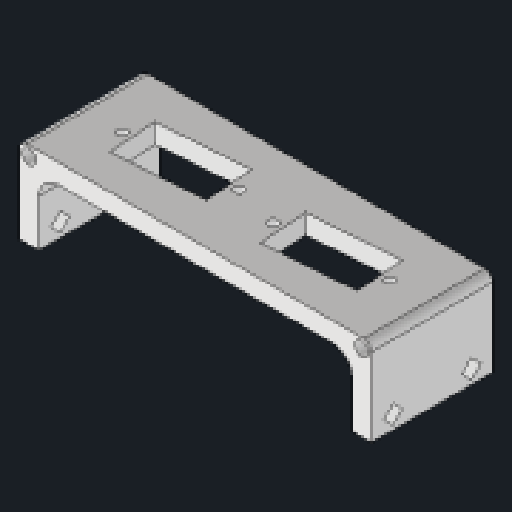
# Autodesk Inventor part: Module Frame
Saved by Autodesk Inventor 2023.2 (Build 272271030, 271C)
## iProperties
Created: 2024-02-26
Part Number: Module Frame
Material: Generic
Document SubType Name: Modeling
Designer: robpl
Density: 1 g/cm^3
Appearance: Default
Author: robpl
Autodesk Inventor part; units mm, degrees
ref_plane "YZ Plane" through (0, 0, 0) normal (1, 0, 0) x (0, 1, 0)
ref_plane "XZ Plane" through (0, 0, 0) normal (0, 1, 0) x (-1, 0, 0)
ref_plane "XY Plane" through (0, 0, 0) normal (0, 0, 1) x (1, 0, 0)
sketch "Sketch1" plane through (0, 0, 0) normal (0, 0, 1) x (1, 0, 0)
  line L0 (-40, 0) -> (40, 0)
  line L1 (40, 0) -> (40, 5)
  line L2 (40, 5) -> (-40, 5)
  line L3 (-40, 5) -> (-40, 0)
  line L4 (-40, 5) -> (-45, 5)
  line L5 (-45, 5) -> (-45, -17)
  line L6 (-45, -17) -> (-40, -17)
  line L7 (-40, -17) -> (-40, 5)
  line L8 (40, 5) -> (45, 5)
  line L9 (45, 5) -> (45, -17)
  line L10 (45, -17) -> (40, -17)
  line L11 (40, -17) -> (40, 5)
  point P0 (0, 0)
  point P1 (0, 0)
  point P2 (40, 0)
  dimension "d0" = 5
  dimension "d1" = 80
  dimension "d2" = 22
  dimension "d11" = 5
  constraints: 24 end point, 6 parallel, 3 horizontal, 3 perpendicular, 2 equal length, 1 coincident, 1 midpoint
  measures "d0" distance of L0.end L1.end
  measures "d1" distance of L0.start L0.end
  measures "d2" distance of L6.end L2.end
  measures "d11" distance of L9.end L10.end
extrude "Extrusion1" add sketch "Sketch1" along normal mid plane 32
sketch "Sketch2" plane through (45, -17, -16) normal (1, 0, 0) x (0, 0, -1)
  line L0 (-28.4042, 3.5) -> (-26, 1.0958)
  line L1 (-26, 1.0958) -> (-23.5958, 3.5)
  line L2 (-23.5958, 3.5) -> (-26, 5.9042)
  line L3 (-26, 5.9042) -> (-28.4042, 3.5)
  line L4 (-28.4042, 3.5) -> (-23.5958, 3.5) construction
  line L5 (-26, 1.0958) -> (-26, 5.9042) construction
  line L6 (-8.4042, 3.5) -> (-6, 1.0958)
  line L7 (-6, 1.0958) -> (-3.5958, 3.5)
  line L8 (-3.5958, 3.5) -> (-6, 5.9042)
  line L9 (-6, 5.9042) -> (-8.4042, 3.5)
  line L10 (-8.4042, 3.5) -> (-3.5958, 3.5) construction
  line L11 (-6, 1.0958) -> (-6, 5.9042) construction
  line L12 (0, 22) -> (-32, 22) projected
  point P0 (-16, 17)
  point P1 (-26, 3.5)
  point P2 (-6, 3.5)
  point P3 (-6, 3.5)
  point P4 (-26, 3.5)
  point P5 (-6, 3.5)
  point P6 (-16, 22)
  point P7 (-26, 3.5)
  dimension "d5" = 3.4
  dimension "d6" = 20
  dimension "d7" = 18.5
  dimension "d8" = 10
  constraints: 24 end point, 9 midpoint, 5 parallel, 5 perpendicular, 1 horizontal, 1 horizontal alignment
  measures "d5" distance of L0.end L1.end
  measures "d6" distance of point (-6, 3.5) point (-26, 3.5)
  measures "d7" distance from line of L12 point (-6, 3.5)
  measures "d8" horizontal distance of point (-16, 22) point (-26, 3.5)
extrude "Extrusion2" cut sketch "Sketch2" against normal through all
sketch "Sketch3" plane through (-45, 0, -16) normal (0, 1, 0) x (1, 0, 0)
  line L0 (39.1905, -14.5) -> (11.4768, -16.689)
  line L1 (50.8095, -17.5) -> (78.5232, -15.311)
  line L2 (0, 0) -> (90, 0) projected
  line L3 (0, 0) -> (0, -32) projected
  line L4 (90, -32) -> (0, -32) projected
  line L5 (90, 0) -> (90, -32) projected
  point P0 (45, -16)
  point P1 (69.8003, -16)
  point P2 (20.1997, -16)
  point P3 (90, -16)
  point P4 (45, -32)
  dimension "d12" = 12
  dimension "d13" = 27.8
  dimension "d14" = 19.05
  dimension "d15" = 19.05
  dimension "d16" = 32
  dimension "d17" = 11.6189
  dimension "d18" = 5.8095
  dimension "d19" = 3
  constraints: 4 end point, 2 horizontal alignment, 2 midpoint, 2 parallel, 2 point on line, 1 coincident
  measures "d12" distance of L0.start L1.start
  measures "d13" distance of L0.start L0.end
  measures "d14" distance of L1.start point (69.8, -16)
  measures "d15" distance of L0.start point (20.2, -16)
  measures "d16" distance of L2.end L4.start
  measures "d17" horizontal distance of L1.start L0.start
  measures "d18" horizontal distance of point (45, -32) L1.start
  measures "d19" vertical distance of L1.start L0.start
hole "Hole1" at (5.8095, 0, 1.5) at (-5.8095, 0, -1.5) at (33.5232, 0, -0.689) at (-33.5232, 0, 0.689) direction (0, 1, 0) diameter 2.5 end through all counterbore diameter 3.7 counterbore depth 4
sketch "Sketch4" plane through (-45, 5, -16) normal (0, 1, 0) x (1, 0, 0)
  line L0 (0, 0) -> (90, 0) projected
  line L1 (0, 0) -> (0, -32) projected
  line L2 (90, -32) -> (0, -32) projected
  line L3 (90, 0) -> (90, -32) projected
  line L4 (78.5232, -15.311) -> (50.8095, -17.5)
  line L5 (39.1905, -14.5) -> (11.4768, -16.689)
  line L6 (76.6227, -21.7306) -> (53.6941, -23.5416)
  line L7 (53.6941, -23.5416) -> (52.7099, -11.0804)
  line L8 (52.7099, -11.0804) -> (75.6385, -9.2694)
  line L9 (75.6385, -9.2694) -> (76.6227, -21.7306)
  line L10 (76.6227, -21.7306) -> (52.7099, -11.0804) construction
  line L11 (53.6941, -23.5416) -> (75.6385, -9.2694) construction
  line L12 (14.3615, -22.7306) -> (37.2901, -20.9196)
  line L13 (37.2901, -20.9196) -> (36.3059, -8.4584)
  line L14 (36.3059, -8.4584) -> (13.3773, -10.2694)
  line L15 (13.3773, -10.2694) -> (14.3615, -22.7306)
  line L16 (14.3615, -22.7306) -> (36.3059, -8.4584) construction
  line L17 (37.2901, -20.9196) -> (13.3773, -10.2694) construction
  circle A0 centre (39.1905, -14.5) radius 1.85 projected
  circle A1 centre (78.5232, -15.311) radius 1.85 projected
  circle A2 centre (50.8095, -17.5) radius 1.85 projected
  circle A3 centre (39.1905, -14.5) radius 1.85 projected
  circle A4 centre (11.4768, -16.689) radius 1.85 projected
  line L18 (85, 0) -> (85, -32) projected
  line L19 (5, -32) -> (85, -32) projected
  line L20 (5, 0) -> (5, -32) projected
  line L21 (85, 0) -> (5, 0) projected
  point P0 (45, -16)
  point P1 (64.6663, -16.4055)
  point P2 (25.3337, -15.5945)
  point P3 (25.3337, -15.5945)
  dimension "d27" = 23
  dimension "d28" = 12.5
  constraints: 28 end point, 8 midpoint, 8 parallel, 4 coincident, 2 perpendicular
  measures "d27" distance of L7.end L8.end
  measures "d28" distance of L6.end L7.end
extrude "Extrusion3" cut sketch "Sketch4" against normal through all contours L9 L6 L7 L4 | L4 L7 L8 L9 | L13 L12 L15 L5 | L5 L15 L14 L13
sketch "Sketch5" plane through (0, 0, -16) normal (0, 0, -1) x (-1, 0, 0)
  line L0 (-45, 5) -> (-45, -17) projected
  line L1 (-45, -17) -> (-40, -17) projected
  line L2 (-40, -17) -> (-40, 0) projected
  line L3 (-40, 0) -> (40, 0) projected
  line L4 (40, 0) -> (40, -17) projected
  line L5 (40, -17) -> (45, -17) projected
  line L6 (45, -17) -> (45, 5) projected
  line L7 (45, 5) -> (-45, 5) projected
  point P0 (0, 0)
  point P1 (-42.5, 2.5)
  point P2 (42.5, 2.5)
  dimension "d31" = 2.5
  dimension "d32" = 2.5
  dimension "d33" = 2.5
  constraints: 1 horizontal alignment
  measures "d31" distance from line of L0 point (-42.5, 2.5)
  measures "d32" distance from line of L7 point (-42.5, 2.5)
  measures "d33" distance from line of L6 point (42.5, 2.5)
hole "Hole2" at (42.5, 2.5, -16) at (-42.5, 2.5, -16) direction (0, 0, 1) diameter 3.7 depth 3.5
mirror "Mirror1" about plane through (0, 0, 0) normal (0, 0, 1) of "Hole2"
fillet "Fillet1" radius 2 2 edges at (-45, 5, 0) (45, 5, 0)
fillet "Fillet2" radius 5 2 edges at (-40, 0, 0) (40, 0, 0)
equation "\"d8\" = 0.5 * d6"
equation "\"d15\" = d14"
equation "\"d18\" = 0.5 * d17"
equation "\"d33\" = d31"
body "Solid1"
